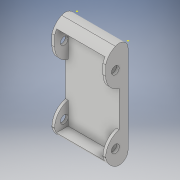
# Autodesk Inventor part: chasis for robot car
Saved by Autodesk Inventor 2019 (Build 230136000, 136)
## iProperties
Created: 2020-12-11
Part Number: chasis for robot car
Material: Generic
Document SubType Name: Modeling
Designer: dennis gordionok
Density: 1 g/cm^3
Appearance: Default
Author: dennis gordionok
Autodesk Inventor part; units mm, degrees
ref_plane "YZ Plane" through (0, 0, 0) normal (1, 0, 0) x (0, 1, 0)
ref_plane "XZ Plane" through (0, 0, 0) normal (0, 1, 0) x (-1, 0, 0)
ref_plane "XY Plane" through (0, 0, 0) normal (0, 0, 1) x (1, 0, 0)
sketch "Sketch1" plane through (0, 0, 0) normal (0, 0, 1) x (1, 0, 0)
  line L0 (-7.6725, 9.18) -> (144.7275, 9.18)
  line L1 (144.7275, 9.18) -> (144.7275, -295.62)
  line L2 (144.7275, -295.62) -> (-7.6725, -295.62)
  line L3 (-7.6725, -295.62) -> (-7.6725, 9.18)
  point P0 (0, 0)
  dimension "d0" = 152.4
  dimension "d1" = 304.8
  constraints: 8 end point, 2 parallel, 1 horizontal, 1 perpendicular
  measures "d0" distance of L1.end L2.end
  measures "d1" distance of L0.end L1.end
extrude "Extrusion1" add sketch "Sketch1" along normal blind 25.4
sketch "Sketch2" plane through (0, 0, 25.4) normal (0, 0, 1) x (1, 0, 0)
  line L0 (144.7275, 9.18) -> (-7.6725, 9.18) projected
  line L1 (-7.6725, 9.18) -> (-7.6725, -26.9908)
  line L2 (-7.6725, 9.18) -> (-7.6725, -295.62) projected
  line L3 (144.7275, -295.62) -> (144.7275, 9.18) projected
  line L4 (144.7275, 9.18) -> (144.7275, -26.9908)
  line L5 (144.7275, -26.9908) -> (-7.6725, -26.9908)
  line L6 (-7.6725, 9.18) -> (144.7275, 9.18)
  point P0 (0, 0)
  constraints: 8 end point, 2 point on line, 1 parallel, 1 perpendicular
extrude "Extrusion2" add sketch "Sketch2" along normal blind 38.1
fillet "Fillet1" radius 50.8 1 edges at (68.5275, 9.18, 63.5)
sketch "Sketch3" plane through (0, 0, 25.4) normal (0, 0, 1) x (1, 0, 0)
  line L0 (-7.6725, -26.9908) -> (-7.6725, -295.62) projected
  line L1 (-7.6725, -26.9908) -> (-7.6725, -104.161)
  line L2 (0, -104.161) -> (0, -26.9908)
  line L3 (0, -26.9908) -> (-7.6725, -26.9908)
  line L4 (0, -104.161) -> (-7.6725, -104.161)
  line L5 (144.7275, -26.9908) -> (-7.6725, -26.9908) projected
  line L6 (144.7275, -26.9908) -> (137.0567, -26.9908)
  line L7 (137.0567, -26.9908) -> (137.0567, -104.161)
  line L8 (137.0567, -104.161) -> (144.7275, -104.161)
  line L9 (144.7275, 9.18) -> (144.7275, -295.62) projected
  line L10 (144.7275, -26.9908) -> (144.7275, -104.161)
  point P0 (0, 0)
  dimension "d7" = 7.6708
  constraints: 16 end point, 5 point on line, 3 perpendicular, 1 parallel, 1 vertical
  measures "d7" distance of L5.start L6.end
extrude "Extrusion3" add sketch "Sketch3" along normal blind 38.1 contours L9 L8 L7 L5
sketch "Sketch4" plane through (0, 0, 25.4) normal (0, 0, 1) x (1, 0, 0)
  line L0 (-7.6725, -26.9908) -> (-7.6725, 9.18) projected
  line L1 (-7.6725, -26.9908) -> (0, -26.9908)
  line L2 (137.0567, -26.9908) -> (-7.6725, -26.9908) projected
  line L3 (-7.6725, -295.62) -> (-7.6725, 9.18) projected
  line L4 (0, -104.9824) -> (-7.6725, -104.9824)
  line L5 (-7.6725, -26.9908) -> (-7.6725, -104.9824)
  line L6 (0, -104.9824) -> (0, -26.9908)
  point P0 (0, 0)
  constraints: 8 end point, 1 collinear, 1 parallel, 1 point on line
extrude "Extrusion4" add sketch "Sketch4" along normal blind 38.1
fillet "Fillet2" radius 50.8 1 edges at (-3.8363, -104.9824, 63.5)
fillet "Fillet3" radius 50.8 1 edges at (140.8921, -104.161, 63.5)
sketch "Sketch5" plane through (137.0567, -26.9908, 25.4) normal (0, -1, 0) x (1, 0, 0)
  line L0 (-137.0567, 38.1) -> (0, 38.1) projected
  line L1 (-137.0567, 38.1) -> (-137.0567, 0) projected
  line L2 (-137.0567, 38.1) -> (-137.0567, 0)
  line L3 (0, 0) -> (-137.0567, 0) projected
  line L4 (-137.0567, 0) -> (0, 0)
  line L5 (0, 0) -> (0, 38.1) projected
  line L6 (0, 0) -> (0, 38.1)
  line L7 (0, 38.1) -> (-137.0567, 38.1)
  point P0 (-137.0567, -25.4)
  constraints: 8 end point, 2 collinear, 2 perpendicular
extrude "Extrusion5" cut sketch "Sketch5" against normal blind 12.7
sketch "Sketch6" plane through (0, 0, 25.4) normal (0, 0, 1) x (1, 0, 0)
  line L0 (-7.6725, -295.62) -> (-7.6725, 9.18) projected
  line L1 (144.7275, -295.62) -> (-7.6725, -295.62)
  line L2 (-7.6725, -295.62) -> (-7.6725, -256.2446)
  line L3 (144.7275, -295.62) -> (144.7275, -256.2446)
  line L4 (144.7275, -295.62) -> (144.7275, -104.161) projected
  line L5 (-7.6725, -256.2446) -> (144.7275, -256.2446)
  point P0 (0, 0)
  constraints: 8 end point, 2 point on line, 1 perpendicular
extrude "Extrusion6" add sketch "Sketch6" along normal blind 38.1
fillet "Fillet4" radius 50.8 1 edges at (68.5275, -295.62, 63.5)
sketch "Sketch7" plane through (0, 0, 25.4) normal (0, 0, 1) x (1, 0, 0)
  line L0 (137.676, -256.2446) -> (144.7275, -256.2446)
  line L1 (-7.6725, -295.62) -> (-7.6725, 9.18) projected
  line L2 (-7.6725, -256.2446) -> (144.7275, -256.2446) projected
  line L3 (-7.6725, -256.2446) -> (-7.6725, -205.4446)
  line L4 (-7.6725, -205.4446) -> (0, -205.4446)
  line L5 (0, -205.4446) -> (0, -256.2446)
  point P0 (0, 0)
  dimension "d20" = 50.8
  constraints: 8 end point, 2 perpendicular, 2 point on line
  measures "d20" distance of L2.start L3.end
extrude "Extrusion7" add sketch "Sketch7" along normal blind 38.1
sketch "Sketch8" plane through (0, 0, 25.4) normal (0, 0, 1) x (1, 0, 0)
  line L0 (0, -256.2446) -> (144.7275, -256.2446) projected
  line L1 (144.7275, -256.2446) -> (144.7275, -205.4446)
  line L2 (144.7275, -256.2446) -> (144.7275, -104.161) projected
  line L3 (144.7275, -205.4446) -> (137.0567, -205.4446)
  line L4 (137.0567, -205.4446) -> (137.0567, -256.2446)
  line L5 (137.0567, -256.2446) -> (144.7275, -256.2446)
  point P0 (0, 0)
  dimension "d23" = 50.8
  dimension "d24" = 7.6708
  constraints: 8 end point, 3 perpendicular, 1 point on line
  measures "d23" distance of L0.end L1.end
  measures "d24" distance of L1.end L3.end
extrude "Extrusion8" add sketch "Sketch8" along normal blind 38.1
fillet "Fillet5" radius 50.8 2 edges at (-3.8363, -205.4446, 63.5) (140.8921, -205.4446, 63.5)
sketch "Sketch9" plane through (0, -256.2446, 63.5) normal (0, 1, 0) x (1, 0, 0)
  line L0 (0, 38.1) -> (137.0567, 38.1) projected
  line L1 (137.0567, 38.1) -> (0, 38.1)
  line L2 (0, 38.1) -> (0, 0) projected
  line L3 (0, 38.1) -> (0, 0)
  line L4 (137.0567, 0) -> (0, 0) projected
  line L5 (0, 0) -> (137.0567, 0)
  line L6 (137.0567, 0) -> (137.0567, 38.1)
  point P0 (0, 63.5)
  constraints: 8 end point, 3 collinear, 1 vertical
extrude "Extrusion9" cut sketch "Sketch9" against normal blind 12.7
sketch "Sketch10" plane through (144.7275, -295.62, 0) normal (1, 0, 0) x (0, 0, -1)
  point P0 (0, 295.62)
fillet "Fillet6" radius 25.4 1 edges at (68.5275, -295.62, 0)
fillet "Fillet7" radius 25.4 1 edges at (68.5275, 9.18, 0)
sketch "Sketch21" plane through (0, 0, 25.4) normal (0, 0, 1) x (1, 0, 0)
  point P0 (0, 0)
sketch "Sketch22" plane through (0, 0, 25.4) normal (0, 0, 1) x (1, 0, 0)
  point P0 (0, 0)
sketch "Sketch23" plane through (0, -55.7956, 63.5) normal (1, 0, 0) x (0, 0, -1)
  point P0 (63.5, 55.7956)
sketch "Sketch24" plane through (0, -55.7956, 63.5) normal (1, 0, 0) x (0, 0, -1)
  circle A0 centre (27.2379, 1.6041) radius 10.8621
  line L0 (38.1, -49.1869) -> (38.1, 41.5047) projected
  point P0 (63.5, 55.7956)
  constraints: 1 centre point, 1 tangent
extrude "Extrusion18" cut sketch "Sketch24" against normal blind 25.4
sketch "Sketch25" plane through (137.0567, -54.9742, 63.5) normal (-1, 0, 0) x (0, 0, 1)
  circle A0 centre (-27.2379, 0.7827) radius 10.8621 projected
  circle A1 centre (-27.2379, 0.7827) radius 10.8621
  point P0 (-63.5, 54.9742)
  constraints: 1 centre point, 1 coincident
extrude "Extrusion19" cut sketch "Sketch25" against normal blind 25.4
sketch "Sketch26" plane through (137.0567, -268.9446, 25.4) normal (-1, 0, 0) x (0, 0, 1)
  circle A0 centre (10.6882, 21.8663) radius 11.2364
  point P0 (-25.4, 268.9446)
  constraints: 1 centre point
extrude "Extrusion20" cut sketch "Sketch26" against normal blind 25.4
sketch "Sketch27" plane through (0, -268.9446, 25.4) normal (1, 0, 0) x (0, 0, -1)
  arc A0 (0, 25.3331) -> (0, 18.3996) centre (-10.6882, 21.8663) ccw projected
  circle A1 centre (-10.6882, 21.8663) radius 11.2364
  point P0 (25.4, 268.9446)
  constraints: 1 centre point, 1 coincident
extrude "Extrusion21" cut sketch "Sketch27" against normal blind 25.4
body "Solid1"
